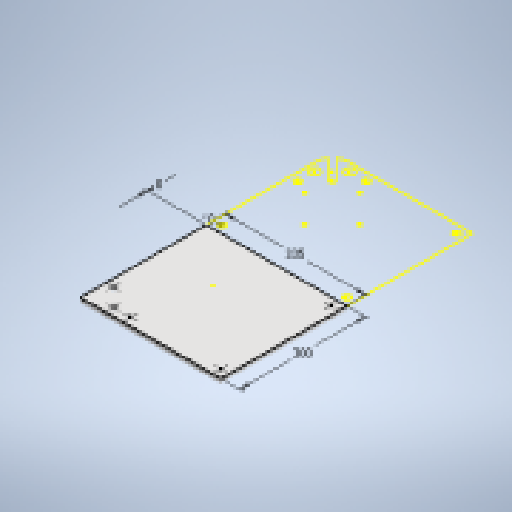
# Autodesk Inventor part: Left bottom plate
Saved by Autodesk Inventor 2024 (Build 280153000, 153)
## iProperties
Created: 2024-03-26
Part Number: Left bottom plate
Material: Generic
Document SubType Name: Modeling
Designer: jens1
Density: 1 g/cm^3
Appearance: Default
Author: jens1
Autodesk Inventor part; units mm, degrees
ref_plane "YZ Plane" through (0, 0, 0) normal (1, 0, 0) x (0, 1, 0)
ref_plane "XZ Plane" through (0, 0, 0) normal (0, 1, 0) x (-1, 0, 0)
ref_plane "XY Plane" through (0, 0, 0) normal (0, 0, 1) x (1, 0, 0)
sketch "Sketch1" plane through (0, 0, 0) normal (0, 1, 0) x (-1, 0, 0)
  line L0 (135.8628, 182.2707) -> (-199.1372, 182.2707)
  line L1 (-199.1372, 182.2707) -> (-199.1372, -117.7293)
  line L2 (-199.1372, -117.7293) -> (135.8628, -117.7293)
  line L3 (135.8628, -117.7293) -> (135.8628, 182.2707)
  circle A0 centre (-46.1372, -301.7293) radius 4.5 projected
  circle A1 centre (19.8628, -367.7293) radius 4.5 projected
  circle A2 centre (19.8628, -235.7293) radius 4.5 projected
  circle A3 centre (85.8628, -301.7293) radius 4.5 projected
  line L4 (83.3404, -354.6002) -> (128.9488, -400.2086) projected
  arc A4 (128.9488, -400.2086) -> (135.8628, -377.7293) centre (95.8628, -377.7293) ccw projected
  line L5 (135.8628, -377.7293) -> (135.8628, -117.7293) projected
  line L6 (135.8628, -117.7293) -> (-199.1372, -117.7293) projected
  line L7 (-199.1372, -117.7293) -> (-199.1372, -417.7293) projected
  line L8 (-199.1372, -417.7293) -> (95.8628, -417.7293) projected
  arc A5 (95.8628, -417.7293) -> (118.3422, -410.8152) centre (95.8628, -377.7293) ccw projected
  line L9 (118.3422, -410.8152) -> (72.7338, -365.2068) projected
  arc A6 (83.3404, -354.6002) -> (72.7338, -365.2068) centre (78.0371, -359.9035) ccw projected
  circle A7 centre (117.0128, -356.8793) radius 11.75 projected
  circle A8 centre (75.0128, -398.8793) radius 11.75 projected
  circle A9 centre (35.4128, -398.8793) radius 7.85 projected
  circle A10 centre (117.0128, -317.2793) radius 7.85 projected
  circle A11 centre (-180.2872, -136.5793) radius 7.85 projected
  circle A12 centre (-180.2872, -398.8793) radius 7.85 projected
  circle A13 centre (117.0128, -136.5793) radius 7.85 projected
  point P0 (0, 0)
  point P1 (117.0128, 121.4207)
  point P2 (75.0128, 163.4207)
  point P3 (35.4128, 163.4207)
  point P4 (-180.2872, -98.8793)
  point P5 (-180.2872, 163.4207)
  point P6 (117.0128, 121.4207)
  point P7 (75.0128, 163.4207)
  point P8 (35.4128, 163.4207)
  point P9 (-180.2872, 163.4207)
  point P10 (-180.2872, -98.8793)
  dimension "d0" = 335
  dimension "d1" = 300
  dimension "d2" = 0
  dimension "d3" = 0
  constraints: 8 end point, 5 coincident, 5 symmetric about line, 2 parallel, 1 horizontal, 1 perpendicular
  measures "d0" distance of L2.end L1.end
  measures "d1" distance of L1.end L0.end
  measures "d2" distance between parallel lines of L6 L2
  measures "d3" distance between parallel lines of L5 L3
extrude "Extrusion1" add sketch "Sketch1" against normal blind 10.5 contours L3 L2 L1 L0
hole "Hole1" at (-117.0128, 0, 121.4207) at (-75.0128, 0, 163.4207) direction (0, -1, 0) diameter 12 end through all countersink diameter 23.5 countersink angle 90
hole "Hole2" at (-35.4128, 0, 163.4207) at (180.2872, 0, 163.4207) at (180.2872, 0, -98.8793) direction (0, -1, 0) diameter 8 end through all countersink diameter 15.7 countersink angle 90
fillet "Fillet1" radius 40 1 edges at (-135.8628, -5.25, 182.2707)
body "Solid1"
